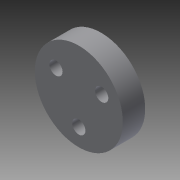
# Autodesk Inventor part: hub
Saved by Autodesk Inventor 2013 (Build 170138000, 138)
## iProperties
Created: 2014-09-26
Part Number: hub
Material: Generic
Document SubType Name: Modeling
Designer: Dan
Density: 1 g/cm^3
Author: Dan
Autodesk Inventor part; units mm, degrees
ref_plane "YZ Plane" through (0, 0, 0) normal (1, 0, 0) x (0, 1, 0)
ref_plane "XZ Plane" through (0, 0, 0) normal (0, 1, 0) x (-1, 0, 0)
ref_plane "XY Plane" through (0, 0, 0) normal (0, 0, 1) x (1, 0, 0)
sketch "Sketch1" plane through (0, 0, 0) normal (0, 1, 0) x (-1, 0, 0)
  circle A0 centre (0, 0) radius 50
  dimension "d0" = 100
  constraints: 1 centre point, 1 coincident
  measures "d0" diameter of A0
extrude "Extrusion1" add sketch "Sketch1" along normal blind 25.4
sketch "Sketch2" plane through (0, 25.4, 0) normal (0, 1, 0) x (1, 0, 0)
  circle A0 centre (0, 0) radius 50 projected
  circle A1 centre (0, 30) radius 7.5
  line L0 (0, 30) -> (0, 0) construction
  dimension "d3" = 15
  dimension "d4" = 30
  constraints: 2 end point, 1 centre point, 1 vertical
  measures "d3" diameter of A1
  measures "d4" distance of L0.start L0.end
extrude "Extrusion3" cut sketch "Sketch2" against normal through all contours A1
pattern_circular "Circular Pattern1" count 3 over 360 about axis through (0, 0, 0) along (0, 1, 0) of "Extrusion3"
body "Solid1"
